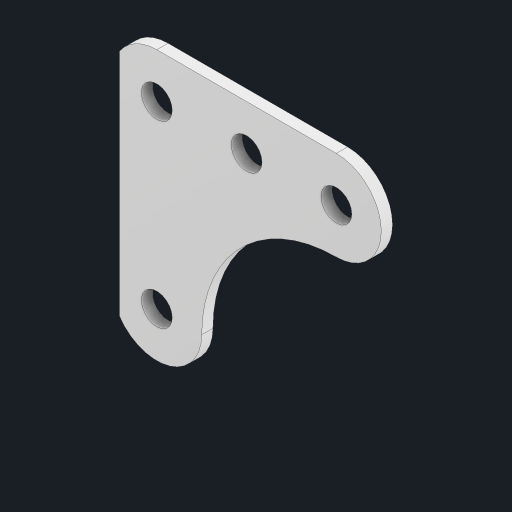
# Autodesk Inventor part: bed_gusset
Saved by Autodesk Inventor 2024 (Build 280153000, 153)
## iProperties
Created: 2023-08-16
Part Number: bed_gusset
Material: Acetal Resin, White
Document SubType Name: Modeling
Designer: avere
Density: 1.425 g/cm^3
Appearance: Smooth - White
Author: avere
Autodesk Inventor part; units mm, degrees
ref_plane "YZ Plane" through (0, 0, 0) normal (1, 0, 0) x (0, 1, 0)
ref_plane "XZ Plane" through (0, 0, 0) normal (0, 1, 0) x (-1, 0, 0)
ref_plane "XY Plane" through (0, 0, 0) normal (0, 0, 1) x (1, 0, 0)
sketch "Sketch1" plane through (0, 0, 0) normal (0, 0, 1) x (1, 0, 0)
  circle A0 centre (-6.536, 14.6455) radius 2.1844
  circle A1 centre (18.864, 14.6455) radius 2.1844
  circle A2 centre (-6.536, -10.7545) radius 2.1844
  circle A3 centre (6.164, 14.6455) radius 2.1844
  arc A4 (-6.536, 20.9955) -> (-11.8124, 18.1785) centre (-6.536, 14.6455) ccw
  arc A5 (18.864, 8.2955) -> (18.864, 20.9955) centre (18.864, 14.6455) ccw
  line L0 (18.864, 20.9955) -> (-6.536, 20.9955)
  line L1 (18.864, 8.2955) -> (18.864, 8.2955)
  arc A6 (-11.8124, -14.2875) -> (-0.186, -10.7545) centre (-6.536, -10.7545) ccw
  line L2 (-0.186, -10.7545) -> (-0.186, -10.7545)
  arc A7 (18.864, 8.2955) -> (-0.186, -10.7545) centre (18.864, -10.7545) ccw
  line L3 (-11.8124, -14.2875) -> (-11.8124, 18.1785)
  point P0 (0, 0)
  point P1 (-0.186, -10.7545)
  dimension "d0" = 4.3688
  dimension "d1" = 4.3688
  dimension "d2" = 4.3688
  dimension "d3" = 4.3688
  dimension "d4" = 12.7
  dimension "d5" = 12.7
  dimension "d6" = 12.7
  dimension "d7" = 19.05
  constraints: 8 centre point, 8 end point, 8 point on circle, 6 tangent, 3 coincident, 1 horizontal, 1 parallel
  measures "d0" diameter of A0
  measures "d1" diameter of A1
  measures "d2" diameter of A2
  measures "d3" diameter of A3
  measures "d4" diameter of A4
  measures "d5" diameter of A5
  measures "d6" diameter of A6
  measures "d7" radius of A7
extrude "Extrusion1" add sketch "Sketch1" along normal blind 1.5875
body "Solid1"
